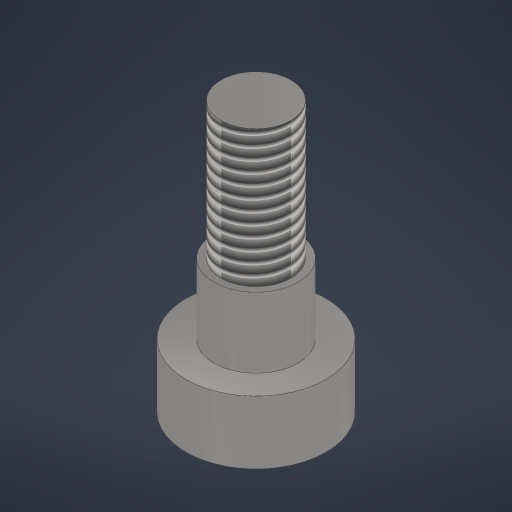
# Autodesk Inventor part: Ali_d6-M5
Saved by Autodesk Inventor 2024.3 (Build 283343000, 343)
## iProperties
Created: 2025-01-09
Part Number: Ali_d6-M5
Material: 스테인리스스틸
Document SubType Name: Modeling
Designer: ASUS
Density: 8 g/cm^3
Appearance: 반연마
Author: ASUS
Autodesk Inventor part; units mm, degrees
ref_plane "YZ Plane" through (0, 0, 0) normal (1, 0, 0) x (0, 1, 0)
ref_plane "XZ Plane" through (0, 0, 0) normal (0, 1, 0) x (-1, 0, 0)
ref_plane "XY Plane" through (0, 0, 0) normal (0, 0, 1) x (1, 0, 0)
sketch "스케치1" plane through (0, 0, 0) normal (0, 0, 1) x (1, 0, 0)
  line L0 (0, 0) -> (0, 20)
  line L1 (0, 0) -> (5, 0)
  line L2 (5, 0) -> (5, 4.5)
  line L3 (5, 4.5) -> (0, 4.5)
  line L4 (0, 4.5) -> (0, 0)
  line L5 (0, 4.5) -> (3, 4.5)
  line L6 (3, 4.5) -> (3, 9.5)
  line L7 (3, 9.5) -> (0, 9.5)
  line L8 (0, 9.5) -> (0, 4.5)
  line L9 (0, 9.5) -> (2.5, 9.5)
  line L10 (2.5, 9.5) -> (2.5, 19.25)
  line L11 (2.5, 19.25) -> (0, 19.25)
  line L12 (0, 19.25) -> (0, 9.5)
  dimension "d0" = 20
  dimension "d1" = 5
  dimension "d2" = 4.5
  dimension "d3" = 3
  dimension "d4" = 5
  dimension "d5" = 2.5
  dimension "d6" = 9.75
  constraints: 26 end point, 6 parallel, 4 perpendicular, 2 point on line, 1 vertical
  measures "d0" distance of L0.start L0.end
  measures "d1" distance of L0.start L1.end
  measures "d2" distance of L2.end L1.end
  measures "d3" distance of L3.end L5.end
  measures "d4" distance of L6.end L5.end
  measures "d5" distance of L7.end L9.end
  measures "d6" distance of L10.end L9.end
revolve "회전1" add sketch "스케치1" angle 360 about axis through (0, 19.25, 0) along (0, -1, 0)
thread "스레드1" size "M5x0.8" class "6g" standard "ANSI Metric M Profile" full length
